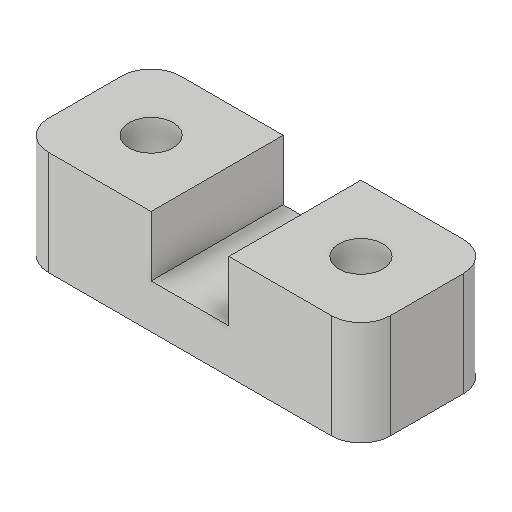
# Autodesk Inventor part: 3DP_PLA_Measurement_Rail_Vibration_Motor_Clamp
Saved by Autodesk Inventor 2026.1 (Build 301233000, 233)
## iProperties
Created: 2018-07-16
Part Number: 3DP_PLA_Measurement_Rail_Vibration_Motor_Clamp
Material: Generic
Document SubType Name: Modeling
Designer: Andrzej
Density: 1 g/cm^3
Appearance: Default
Author: Andrzej
Autodesk Inventor part; units mm, degrees
ref_plane "YZ Plane" through (0, 0, 0) normal (1, 0, 0) x (0, 1, 0)
ref_plane "XZ Plane" through (0, 0, 0) normal (0, 1, 0) x (-1, 0, 0)
ref_plane "XY Plane" through (0, 0, 0) normal (0, 0, 1) x (1, 0, 0)
sketch "Sketch1" plane through (0, 0, 0) normal (0, 0, 1) x (1, 0, 0)
  line L0 (-4.3298, 0.4357) -> (0.9702, 0.4357)
  line L1 (0.9702, 0.4357) -> (0.9702, 4.5357)
  line L2 (-4.3298, 0.4357) -> (-4.3298, 4.5357)
  line L3 (-4.3298, 4.5357) -> (-13.3298, 4.5357)
  line L4 (0.9702, 4.5357) -> (9.9702, 4.5357)
  line L5 (-13.3298, 4.5357) -> (-13.3298, -2.5643)
  line L6 (-13.3298, -2.5643) -> (9.9702, -2.5643)
  line L7 (9.9702, -2.5643) -> (9.9702, 4.5357)
  point P0 (0, 0)
  dimension "d0" = 5.3
  dimension "d1" = 4.1
  dimension "d2" = 9
  dimension "d3" = 9
  dimension "d4" = 3
  dimension "d5" = 4.1
  constraints: 16 end point, 4 perpendicular, 2 horizontal, 2 vertical
  measures "d0" distance of L0.start L0.end
  measures "d1" distance of L0.end L1.end
  measures "d2" distance of L2.end L3.end
  measures "d3" distance of L1.end L4.end
  measures "d4" distance between parallel lines of L6 L0
  measures "d5" distance between parallel lines of L3 L0
extrude "Extrusion1" add sketch "Sketch1" along normal blind 9
sketch "Sketch2" plane through (-13.3298, 4.5357, 0) normal (0, 1, 0) x (1, 0, 0)
  line L0 (0, 0) -> (9, 0) projected
  line L1 (0, 0) -> (0, -9) projected
  line L2 (9, -9) -> (0, -9) projected
  line L3 (9, 0) -> (9, -9) projected
  line L4 (14.3, 0) -> (23.3, 0) projected
  line L5 (14.3, 0) -> (14.3, -9) projected
  line L6 (23.3, -9) -> (14.3, -9) projected
  line L7 (23.3, 0) -> (23.3, -9) projected
  point P0 (13.3298, 0)
  point P1 (4.5, -4.5)
  point P2 (18.8, -4.5)
  dimension "d8" = 9
  dimension "d9" = 9
  dimension "d10" = 4.5
  dimension "d11" = 4.5
  dimension "d12" = 4.5
  dimension "d13" = 4.5
  measures "d8" distance of L0.start L0.end
  measures "d9" distance of L0.start L1.end
  measures "d10" distance from line of L1 point (4.5, -4.5)
  measures "d11" distance from line of L0 point (4.5, -4.5)
  measures "d12" distance from line of L4 point (18.8, -4.5)
  measures "d13" distance from line of L7 point (18.8, -4.5)
hole "Hole1" at (-8.8298, 4.5357, 4.5) at (5.4702, 4.5357, 4.5) direction (0, -1, 0) diameter 3 end through all
fillet "Fillet1" radius 2 4 edges at (-13.3298, 0.9857, 9) (-13.3298, 0.9857, 0) (9.9702, 0.9857, 0) (9.9702, 0.9857, 9)
equation "\"d5\" = d1"
equation "\"d12\" = d11"
equation "\"d13\" = d10"
body "Solid1"
